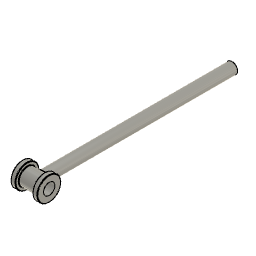
Hydraulic Piston short (Autodesk Fusion 360 design; units mm, degrees)
Autodesk Fusion 360 part; units mm, degrees
sketch "Sketch1" plane through (0, 4.0146, 0) normal (0, -1, 0) x (1, 0, 0)
  circle A0 centre (0, 14.2852) radius 1.18
  circle A1 centre (0, 14.2852) radius 1.2
  dimension "d81" = 2.36
  constraint concentric A0 A1
  measures "d81" diameter of A0
extrude "Extrude1" add sketch "Sketch1" along normal blind 40 contours A0
sketch "Sketch2" plane through (0, 0, 0) normal (1, 0, 0) x (0, 1, 0)
  circle A0 centre (-37.1886, 14.2852) radius 1.8
  circle A1 centre (-37.1886, 14.2852) radius 2.5
  point P0 (-35.9854, 14.2852)
  dimension "d84" = 3.6
  dimension "d85" = 5
  constraint horizontal A0.centre P0
  constraint concentric A0 A1
  measures "d84" diameter of A0
  measures "d85" diameter of A1
extrude "Extrude2" add sketch "Sketch2" along normal mid plane 3.6 contours A0
extrude "Extrude3" add sketch "Sketch2" along normal blind 1 from surface at 1.8 contours A0 | A1
mirror "Mirror1" about plane through (0, 0, 0) normal (1, 0, 0) of "Extrude3"
fillet "Fillet1" radius 0.1 6 edges at (-2.8, -39.5194, 13.3811) (-1.8, -39.5194, 13.3811) (-1.8, -38.8668, 14.9361) (1.8, -38.8668, 13.6342) (1.8, -39.5194, 13.3811) (2.8, -39.5194, 13.3811)
sketch "Sketch3" plane through (2.8, 0, 0) normal (1, 0, 0) x (0, 1, 0)
  circle A0 centre (-37.1886, 14.2852) radius 1.2
  circle A1 centre (-37.1886, 14.2852) radius 2.4
  dimension "d93" = 2.4
  constraint concentric A0 A1
  measures "d93" diameter of A0
extrude "Extrude4" cut sketch "Sketch3" against normal through all contours A0
fillet "Fillet2" radius 0.2 1 edges at (0, -35.8294, 15.4652)
